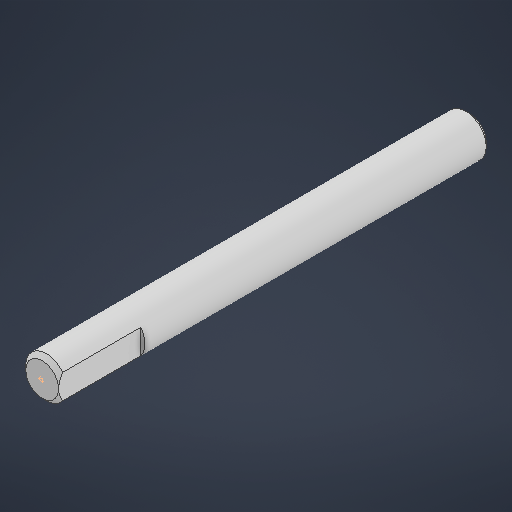
# Autodesk Inventor part: Flywheelshaft
Saved by Autodesk Inventor 2025.4 (Build 294407000, 407)
## iProperties
Created: 2026-05-29
Part Number: Flywheelshaft
Material: Generic
Document SubType Name: Modeling
Designer: VuQuan
Density: 1 g/cm^3
Appearance: Default
Author: VuQuan
Autodesk Inventor part; units mm, degrees
ref_plane "YZ Plane" through (0, 0, 0) normal (1, 0, 0) x (0, 1, 0)
ref_plane "XZ Plane" through (0, 0, 0) normal (0, 1, 0) x (-1, 0, 0)
ref_plane "XY Plane" through (0, 0, 0) normal (0, 0, 1) x (1, 0, 0)
sketch "Sketch1" plane through (0, 0, 0) normal (0, 0, 1) x (1, 0, 0)
  circle A0 centre (0, 0) radius 2.5
  line L0 (2, 1.5) -> (2, -1.5)
  dimension "d0" = 5
  dimension "d1" = 2
  constraints: 2 end point, 2 point on circle, 1 centre point, 1 coincident, 1 vertical
  measures "d0" diameter of A0
  measures "d1" distance from line of point (0, 0) L0
extrude "Extrusion1" add sketch "Sketch1" against normal blind 52
extrude "Extrusion2" cut sketch "Sketch1" against normal blind 10 contours A0 L0 picked at (2.0912, -0.3466)
chamfer "Chamfer1" distance 0.5 angle 45 2 edges at (-2.5, 0, 0) (-2.5, 0, -52)
body "Solid1"
